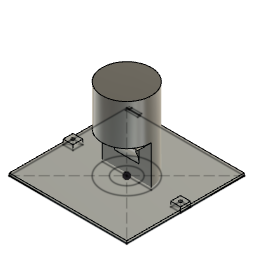
Minecraft Lamp (150x150mm) v6 (Autodesk Fusion 360 design; units mm, degrees)
Autodesk Fusion 360 part; units mm, degrees
sketch "Shade - Vertical Projection" plane through (0, 0, 0) normal (0, 0, 1) x (1, 0, 0) in component "Lamp Shade"
  line L0 (-75, 75) -> (75, 75)
  line L1 (75, 75) -> (75, -75)
  line L2 (75, -75) -> (-75, -75)
  line L3 (-75, -75) -> (-75, 75)
  line L4 (-75, 75) -> (75, -75) construction
  line L5 (75, 75) -> (-75, -75) construction
  line L6 (-72, 72) -> (72, 72)
  line L7 (72, 72) -> (72, -72)
  line L8 (72, -72) -> (-72, -72)
  line L9 (-72, -72) -> (-72, 72)
  line L10 (-72, 72) -> (72, -72) construction
  line L11 (72, 72) -> (-72, -72) construction
  line L12 (-66, 72) -> (-72, 72) construction
  line L13 (-72, 72) -> (-72, 75) construction
  line L14 (-72, 75) -> (-66, 75) construction
  line L15 (-66, 75) -> (-66, 72)
  line L16 (-75, 75) -> (-72, 75) construction
  line L17 (-72, 75) -> (-72, 72) construction
  line L18 (-72, 72) -> (-75, 72) construction
  line L19 (-75, 72) -> (-75, 75) construction
  line L20 (-54, 72) -> (-66, 72)
  line L21 (-66, 72) -> (-66, 75) construction
  line L22 (-66, 75) -> (-54, 75)
  line L23 (-54, 75) -> (-54, 72)
  line L24 (-72, 6) -> (-60, 6)
  line L25 (-60, 6) -> (-60, -6)
  line L26 (-60, -6) -> (-72, -6)
  line L27 (-72, -6) -> (-72, 6)
  line L28 (60, 6) -> (72, 6)
  line L29 (72, 6) -> (72, -6)
  line L30 (72, -6) -> (60, -6)
  line L31 (60, -6) -> (60, 6)
  dimension "d13" = 150
  dimension "d14" = 150
  dimension "d16" = 144
  dimension "d17" = 144
  dimension "d29" = 6
  dimension "d30" = 3
  dimension "d31" = 3
  dimension "d32" = 3
  dimension "d33" = 12
  dimension "d34" = 3
  dimension "d157" = 12
  dimension "d158" = 12
  dimension "d159" = 12
  dimension "d160" = 12
  constraint horizontal L0
  constraint perpendicular L0 L1
  constraint parallel L0 L2
  constraint parallel L1 L3
  constraint coincident L4 origin
  constraint coincident L5 origin
  constraint horizontal L6
  constraint perpendicular L6 L7
  constraint parallel L6 L8
  constraint parallel L7 L9
  constraint coincident L10 origin
  constraint coincident L11 origin
  constraint horizontal L12
  constraint vertical L13
  constraint horizontal L14
  constraint vertical L15
  constraint horizontal L16
  constraint vertical L17
  constraint horizontal L18
  constraint vertical L19
  constraint midpoint L13 L17
  constraint horizontal L20
  constraint vertical L21
  constraint horizontal L22
  constraint vertical L23
  constraint midpoint L15 L21
  constraint horizontal L24
  constraint vertical L25
  constraint horizontal L26
  constraint vertical L27
  constraint midpoint L9 L27
  constraint horizontal L28
  constraint vertical L29
  constraint horizontal L30
  constraint vertical L31
  constraint midpoint L7 L29
  measures "d13" distance of L1.end L2.end
  measures "d14" distance of L0.end L1.end
  measures "d16" distance of L7.end L8.end
  measures "d17" distance of L6.end L7.end
  measures "d29" distance of L12.start L6.start
  measures "d30" distance of L12.start L14.end
  measures "d31" distance of L0.start L13.end
  measures "d32" distance of L0.start L18.end
  measures "d33" distance of L20.start L12.start
  measures "d34" distance of L20.start L22.end
  measures "d157" distance of L24.start L24.end
  measures "d158" distance of L24.start L26.end
  measures "d159" distance of L28.start L28.end
  measures "d160" distance of L28.start L30.end
extrude "Extrude3" add sketch "Shade - Vertical Projection" along normal blind 150 contours L0 L1 L2 L3 L6 L7 L8 L9 L15 L23 L27 L29 | L0 L6 L15 L20 L22 L23 makes body 1 in component "Lamp Shade"
box "BoxPrimitive2" add length 150 width 150 height -3 placed x (0, 1, 0) y (-1, 0, 0) z (0, 0, 1) at (75, -75, 150) bodies 1 in component "Lamp Shade"
sketch "Shade - Back - Holes" plane through (0, 75, 0) normal (0, 1, 0) x (-1, 0, 0) in component "Lamp Shade"
  line L0 (-75, 150) -> (-75, 0)
  line L1 (-75, 0) -> (75, 0)
  line L2 (75, 0) -> (75, 150)
  line L3 (75, 150) -> (-75, 150)
  line L4 (75, 0) -> (69, 0)
  line L5 (69, 0) -> (69, 27) construction
  line L6 (69, 27) -> (75, 27) construction
  line L7 (75, 27) -> (75, 0)
  line L8 (69, 0) -> (57, 0)
  line L9 (57, 0) -> (57, 27)
  line L10 (57, 27) -> (69, 27) construction
  line L11 (69, 27) -> (69, 0)
  line L12 (57, 0) -> (30, 0)
  line L13 (30, 0) -> (30, 27) construction
  line L14 (30, 27) -> (57, 27) construction
  line L15 (57, 27) -> (57, 0) construction
  line L16 (69, 27) -> (57, 0) construction
  line L17 (69, 0) -> (57, 27) construction
  line L18 (57, 27) -> (30, 0) construction
  line L19 (30, 27) -> (57, 0) construction
  circle A0 centre (63, 13.5) radius 6
  circle A1 centre (43.5, 13.5) radius 7.5
  line L20 (69, 0) -> (57, 0)
  line L21 (57, 0) -> (57, 13.5)
  line L22 (57, 13.5) -> (69, 13.5)
  line L23 (69, 13.5) -> (69, 0)
  point P0 (75, 0)
  dimension "d61" = 6
  dimension "d62" = 27
  dimension "d63" = 12
  dimension "d64" = 27
  dimension "d65" = 27
  dimension "d66" = 27
  dimension "d67" = 12
  dimension "d68" = 15
  dimension "d69" = 12
  dimension "d70" = 13.5
  constraint horizontal L4
  constraint vertical L5
  constraint horizontal L6
  constraint vertical L7
  constraint coincident P0 L1.end
  constraint horizontal L8
  constraint vertical L9
  constraint horizontal L10
  constraint vertical L11
  constraint horizontal L12
  constraint vertical L13
  constraint horizontal L14
  constraint vertical L15
  constraint midpoint L17 A0.centre
  constraint midpoint L19 A1.centre
  constraint horizontal L20
  constraint vertical L21
  constraint horizontal L22
  constraint vertical L23
  constraint midpoint L8 L20
  measures "d61" distance of P0 L4.end
  measures "d62" distance of P0 L6.end
  measures "d63" distance of L4.end L8.end
  measures "d64" distance of L4.end L5.end
  measures "d65" distance of L8.end L12.end
  measures "d66" distance of L8.end L9.end
  measures "d67" diameter of A0
  measures "d68" diameter of A1
  measures "d69" distance of L4.end L8.end
  measures "d70" distance of L4.end L22.end
extrude "Extrude5" cut sketch "Shade - Back - Holes" against normal blind 3 contours L1 L8 L9 L11 A0 L20 L21 L23 | A0 L22 | A0 L22 | A1 bodies 1 in component "Lamp Shade"
sketch "Shade - Left" plane through (-75, 0, 0) normal (-1, 0, 0) x (0, -1, 0) in component "Lamp Shade"
  line L0 (-75, 150) -> (-75, 0)
  line L1 (-75, 0) -> (75, 0)
  line L2 (75, 0) -> (75, 150)
  line L3 (75, 150) -> (-75, 150)
  line L4 (-75, 150) -> (75, 150)
  line L5 (75, 150) -> (75, 0)
  line L6 (75, 0) -> (-75, 0)
  line L7 (-75, 0) -> (-75, 150)
  line L8 (75, 0) -> (-75, 0)
  line L9 (-64.2857, 0) -> (-64.2857, 150)
  line L10 (-53.5714, 0) -> (-53.5714, 150)
  line L11 (-42.8571, 0) -> (-42.8571, 150)
  line L12 (-32.1429, 0) -> (-32.1429, 150)
  line L13 (-21.4286, 0) -> (-21.4286, 150)
  line L14 (-10.7143, 0) -> (-10.7143, 150)
  line L15 (0, 0) -> (0, 150)
  line L16 (10.7143, 0) -> (10.7143, 150)
  line L17 (21.4286, 0) -> (21.4286, 150)
  line L18 (32.1429, 0) -> (32.1429, 150)
  line L19 (42.8571, 0) -> (42.8571, 150)
  line L20 (53.5714, 0) -> (53.5714, 150)
  line L21 (64.2857, 0) -> (64.2857, 150)
  line L22 (75, 0) -> (75, 150)
  line L23 (75, 10.7143) -> (-75, 10.7143)
  line L24 (75, 21.4286) -> (-75, 21.4286)
  line L25 (75, 32.1429) -> (-75, 32.1429)
  line L26 (75, 42.8571) -> (-75, 42.8571)
  line L27 (75, 53.5714) -> (-75, 53.5714)
  line L28 (75, 64.2857) -> (-75, 64.2857)
  line L29 (75, 75) -> (-75, 75)
  line L30 (75, 85.7143) -> (-75, 85.7143)
  line L31 (75, 96.4286) -> (-75, 96.4286)
  line L32 (75, 107.1429) -> (-75, 107.1429)
  line L33 (75, 117.8571) -> (-75, 117.8571)
  line L34 (75, 128.5714) -> (-75, 128.5714)
  line L35 (75, 139.2857) -> (-75, 139.2857)
  line L36 (75, 150) -> (-75, 150)
  dimension "d73" = 150
  dimension "d74" = 150
  dimension "d77" = 150
  dimension "d78" = 0
  dimension "d81" = 0
  dimension "d82" = 150
  constraint horizontal L4
  constraint vertical L5
  constraint horizontal L6
  constraint vertical L7
  constraint midpoint L6 L8
  measures "d73" distance of L0.start L2.end
  measures "d74" distance of L0.start L0.end
sketch "Shade - Front" plane through (0, -75, 0) normal (0, -1, 0) x (1, 0, 0) in component "Lamp Shade"
  line L0 (-75, 150) -> (-75, 0)
  line L1 (-75, 0) -> (75, 0)
  line L2 (75, 0) -> (75, 150)
  line L3 (75, 150) -> (-75, 150)
  line L4 (-75, 150) -> (75, 150)
  line L5 (75, 150) -> (75, 0)
  line L6 (75, 0) -> (-75, 0)
  line L7 (-75, 0) -> (-75, 150)
  line L8 (75, 0) -> (-75, 0)
  line L9 (75, 10.7143) -> (-75, 10.7143)
  line L10 (75, 21.4286) -> (-75, 21.4286)
  line L11 (75, 32.1429) -> (-75, 32.1429)
  line L12 (75, 42.8571) -> (-75, 42.8571)
  line L13 (75, 53.5714) -> (-75, 53.5714)
  line L14 (75, 64.2857) -> (-75, 64.2857)
  line L15 (75, 75) -> (-75, 75)
  line L16 (75, 85.7143) -> (-75, 85.7143)
  line L17 (75, 96.4286) -> (-75, 96.4286)
  line L18 (75, 107.1429) -> (-75, 107.1429)
  line L19 (75, 117.8571) -> (-75, 117.8571)
  line L20 (75, 128.5714) -> (-75, 128.5714)
  line L21 (75, 139.2857) -> (-75, 139.2857)
  line L22 (75, 150) -> (-75, 150)
  line L23 (-64.2857, 0) -> (-64.2857, 150)
  line L24 (-53.5714, 0) -> (-53.5714, 150)
  line L25 (-42.8571, 0) -> (-42.8571, 150)
  line L26 (-32.1429, 0) -> (-32.1429, 150)
  line L27 (-21.4286, 0) -> (-21.4286, 150)
  line L28 (-10.7143, 0) -> (-10.7143, 150)
  line L29 (0, 0) -> (0, 150)
  line L30 (10.7143, 0) -> (10.7143, 150)
  line L31 (21.4286, 0) -> (21.4286, 150)
  line L32 (32.1429, 0) -> (32.1429, 150)
  line L33 (42.8571, 0) -> (42.8571, 150)
  line L34 (53.5714, 0) -> (53.5714, 150)
  line L35 (64.2857, 0) -> (64.2857, 150)
  line L36 (75, 0) -> (75, 150)
  line L37 (-75, 150) -> (75, 0) construction
  line L38 (75, 150) -> (-75, 0) construction
  dimension "d83" = 150
  dimension "d84" = 150
  dimension "d87" = 0
  dimension "d88" = 150
  dimension "d91" = 150
  dimension "d92" = 0
  constraint horizontal L4
  constraint vertical L5
  constraint horizontal L6
  constraint vertical L7
  constraint midpoint L6 L8
  constraint coincident L1.end L2.start
  constraint coincident L0.end L1.start
  measures "d83" distance of L0.start L2.end
  measures "d84" distance of L0.start L0.end
sketch "Shade - Right" plane through (75, 0, 0) normal (1, 0, 0) x (0, 1, 0) in component "Lamp Shade"
  line L0 (-75, 150) -> (-75, 0)
  line L1 (-75, 0) -> (75, 0)
  line L2 (75, 0) -> (75, 150)
  line L3 (75, 150) -> (-75, 150)
  line L4 (-75, 150) -> (75, 150)
  line L5 (75, 150) -> (75, 0)
  line L6 (75, 0) -> (-75, 0)
  line L7 (-75, 0) -> (-75, 150)
  line L8 (75, 0) -> (-75, 0)
  line L9 (-64.2857, 0) -> (-64.2857, 150)
  line L10 (-53.5714, 0) -> (-53.5714, 150)
  line L11 (-42.8571, 0) -> (-42.8571, 150)
  line L12 (-32.1429, 0) -> (-32.1429, 150)
  line L13 (-21.4286, 0) -> (-21.4286, 150)
  line L14 (-10.7143, 0) -> (-10.7143, 150)
  line L15 (0, 0) -> (0, 150)
  line L16 (10.7143, 0) -> (10.7143, 150)
  line L17 (21.4286, 0) -> (21.4286, 150)
  line L18 (32.1429, 0) -> (32.1429, 150)
  line L19 (42.8571, 0) -> (42.8571, 150)
  line L20 (53.5714, 0) -> (53.5714, 150)
  line L21 (64.2857, 0) -> (64.2857, 150)
  line L22 (75, 0) -> (75, 150)
  line L23 (75, 10.7143) -> (-75, 10.7143)
  line L24 (75, 21.4286) -> (-75, 21.4286)
  line L25 (75, 32.1429) -> (-75, 32.1429)
  line L26 (75, 42.8571) -> (-75, 42.8571)
  line L27 (75, 53.5714) -> (-75, 53.5714)
  line L28 (75, 64.2857) -> (-75, 64.2857)
  line L29 (75, 75) -> (-75, 75)
  line L30 (75, 85.7143) -> (-75, 85.7143)
  line L31 (75, 96.4286) -> (-75, 96.4286)
  line L32 (75, 107.1429) -> (-75, 107.1429)
  line L33 (75, 117.8571) -> (-75, 117.8571)
  line L34 (75, 128.5714) -> (-75, 128.5714)
  line L35 (75, 139.2857) -> (-75, 139.2857)
  line L36 (75, 150) -> (-75, 150)
  dimension "d93" = 150
  dimension "d94" = 150
  dimension "d97" = 150
  dimension "d98" = 0
  dimension "d101" = 0
  dimension "d102" = 150
  constraint horizontal L4
  constraint vertical L5
  constraint horizontal L6
  constraint vertical L7
  constraint midpoint L6 L8
  measures "d93" distance of L0.start L2.end
  measures "d94" distance of L0.start L0.end
sketch "Shade - Back" plane through (0, 75, 0) normal (0, 1, 0) x (-1, 0, 0) in component "Lamp Shade"
  line L0 (57, 0) -> (57, 13.5)
  arc A0 (69, 13.5) -> (57, 13.5) centre (63, 13.5) ccw
  line L1 (69, 13.5) -> (69, 0)
  line L2 (69, 0) -> (75, 0)
  line L3 (75, 0) -> (75, 150)
  line L4 (75, 150) -> (-75, 150)
  line L5 (-75, 150) -> (-75, 0)
  line L6 (-75, 0) -> (57, 0)
  circle A1 centre (43.5, 13.5) radius 7.5
  line L7 (-75, 150) -> (75, 150)
  line L8 (75, 150) -> (75, 0)
  line L9 (75, 0) -> (-75, 0)
  line L10 (-75, 0) -> (-75, 150)
  line L11 (75, 0) -> (-75, 0)
  line L12 (75, 10.7143) -> (-75, 10.7143)
  line L13 (75, 21.4286) -> (-75, 21.4286)
  line L14 (75, 32.1429) -> (-75, 32.1429)
  line L15 (75, 42.8571) -> (-75, 42.8571)
  line L16 (75, 53.5714) -> (-75, 53.5714)
  line L17 (75, 64.2857) -> (-75, 64.2857)
  line L18 (75, 75) -> (-75, 75)
  line L19 (75, 85.7143) -> (-75, 85.7143)
  line L20 (75, 96.4286) -> (-75, 96.4286)
  line L21 (75, 107.1429) -> (-75, 107.1429)
  line L22 (75, 117.8571) -> (-75, 117.8571)
  line L23 (75, 128.5714) -> (-75, 128.5714)
  line L24 (75, 139.2857) -> (-75, 139.2857)
  line L25 (75, 150) -> (-75, 150)
  line L26 (-64.2857, 0) -> (-64.2857, 150)
  line L27 (-53.5714, 0) -> (-53.5714, 150)
  line L28 (-42.8571, 0) -> (-42.8571, 150)
  line L29 (-32.1429, 0) -> (-32.1429, 150)
  line L30 (-21.4286, 0) -> (-21.4286, 150)
  line L31 (-10.7143, 0) -> (-10.7143, 150)
  line L32 (0, 0) -> (0, 150)
  line L33 (10.7143, 0) -> (10.7143, 150)
  line L34 (21.4286, 0) -> (21.4286, 150)
  line L35 (32.1429, 0) -> (32.1429, 150)
  line L36 (42.8571, 0) -> (42.8571, 150)
  line L37 (53.5714, 0) -> (53.5714, 150)
  line L38 (64.2857, 0) -> (64.2857, 150)
  line L39 (75, 0) -> (75, 150)
  dimension "d103" = 150
  dimension "d104" = 150
  dimension "d107" = 0
  dimension "d108" = 150
  dimension "d111" = 150
  dimension "d112" = 0
  constraint horizontal L7
  constraint vertical L8
  constraint horizontal L9
  constraint vertical L10
  constraint midpoint L9 L11
  measures "d103" distance of L4.end L3.end
  measures "d104" distance of L4.end L5.end
sketch "Shade - Top" plane through (0, 0, 150) normal (0, 0, 1) x (-1, 0, 0) in component "Lamp Shade"
  line L0 (75, 75) -> (-75, 75)
  line L1 (-75, 75) -> (-75, -75)
  line L2 (-75, -75) -> (75, -75)
  line L3 (75, -75) -> (75, 75)
  line L4 (-75, -75) -> (75, -75)
  line L5 (75, -75) -> (75, 75)
  line L6 (75, 75) -> (-75, 75)
  line L7 (-75, 75) -> (-75, -75)
  line L8 (75, 75) -> (-75, 75)
  line L9 (-64.2857, 75) -> (-64.2857, -75)
  line L10 (-53.5714, 75) -> (-53.5714, -75)
  line L11 (-42.8571, 75) -> (-42.8571, -75)
  line L12 (-32.1429, 75) -> (-32.1429, -75)
  line L13 (-21.4286, 75) -> (-21.4286, -75)
  line L14 (-10.7143, 75) -> (-10.7143, -75)
  line L15 (0, 75) -> (0, -75)
  line L16 (10.7143, 75) -> (10.7143, -75)
  line L17 (21.4286, 75) -> (21.4286, -75)
  line L18 (32.1429, 75) -> (32.1429, -75)
  line L19 (42.8571, 75) -> (42.8571, -75)
  line L20 (53.5714, 75) -> (53.5714, -75)
  line L21 (64.2857, 75) -> (64.2857, -75)
  line L22 (75, 75) -> (75, -75)
  line L23 (75, 64.2857) -> (-75, 64.2857)
  line L24 (75, 53.5714) -> (-75, 53.5714)
  line L25 (75, 42.8571) -> (-75, 42.8571)
  line L26 (75, 32.1429) -> (-75, 32.1429)
  line L27 (75, 21.4286) -> (-75, 21.4286)
  line L28 (75, 10.7143) -> (-75, 10.7143)
  line L29 (75, 0) -> (-75, 0)
  line L30 (75, -10.7143) -> (-75, -10.7143)
  line L31 (75, -21.4286) -> (-75, -21.4286)
  line L32 (75, -32.1429) -> (-75, -32.1429)
  line L33 (75, -42.8571) -> (-75, -42.8571)
  line L34 (75, -53.5714) -> (-75, -53.5714)
  line L35 (75, -64.2857) -> (-75, -64.2857)
  line L36 (75, -75) -> (-75, -75)
  dimension "d113" = 150
  dimension "d114" = 150
  dimension "d117" = 150
  dimension "d118" = 0
  dimension "d121" = 0
  constraint horizontal L4
  constraint vertical L5
  constraint horizontal L6
  constraint vertical L7
  constraint midpoint L6 L8
  measures "d113" distance of L1.end L2.end
  measures "d114" distance of L1.end L0.end
sketch "Base - Vertical Projection" plane through (0, 0, 0) normal (0, 0, 1) x (1, 0, 0) in component "Lamp Base"
  line L0 (-72, 72) -> (72, 72)
  line L1 (72, 72) -> (72, -72)
  line L2 (72, -72) -> (-72, -72)
  line L3 (-72, -72) -> (-72, 72)
  line L4 (-72, 72) -> (72, -72) construction
  line L5 (72, 72) -> (-72, -72) construction
  line L6 (-72, 72) -> (-69, 72)
  line L7 (-69, 72) -> (-69, 75)
  line L8 (-69, 75) -> (-72, 75) construction
  line L9 (-72, 75) -> (-72, 72) construction
  line L10 (-57, 72) -> (-69, 72)
  line L11 (-69, 72) -> (-69, 75)
  line L12 (-69, 75) -> (-57, 75)
  line L13 (-57, 75) -> (-57, 72)
  line L14 (-55.5, 69) -> (-70.5, 69)
  line L15 (-70.5, 69) -> (-70.5, 72)
  line L16 (-70.5, 72) -> (-55.5, 72)
  line L17 (-55.5, 72) -> (-55.5, 69)
  line L18 (-60, -6) -> (-72, -6)
  line L19 (-72, -6) -> (-72, 6)
  line L20 (-72, 6) -> (-60, 6)
  line L21 (-60, 6) -> (-60, -6)
  line L22 (72, -6) -> (60, -6)
  line L23 (60, -6) -> (60, 6)
  line L24 (60, 6) -> (72, 6)
  line L25 (72, 6) -> (72, -6)
  line L26 (-60, -6) -> (-72, 6) construction
  line L27 (-72, -6) -> (-60, 6) construction
  line L28 (60, -6) -> (72, 6) construction
  line L29 (72, -6) -> (60, 6) construction
  circle A0 centre (0, 0) radius 30
  circle A1 centre (0, 0) radius 15
  line L30 (0, 0) -> (-30, 0)
  line L31 (0, 0) -> (30, 0)
  dimension "d123" = 144
  dimension "d124" = 144
  dimension "d125" = 3
  dimension "d126" = 3
  dimension "d127" = 12
  dimension "d128" = 3
  dimension "d129" = 15
  dimension "d130" = 3
  dimension "d131" = 12
  dimension "d132" = 12
  dimension "d133" = 12
  dimension "d134" = 12
  dimension "d154" = 60
  dimension "d176" = 30
  constraint horizontal L0
  constraint perpendicular L0 L1
  constraint parallel L0 L2
  constraint parallel L1 L3
  constraint coincident L4 A0.centre
  constraint coincident L5 A0.centre
  constraint coincident A0.centre A1.centre
  constraint horizontal L6
  constraint vertical L7
  constraint horizontal L8
  constraint vertical L9
  constraint horizontal L10
  constraint vertical L11
  constraint horizontal L12
  constraint vertical L13
  constraint midpoint L7 L11
  constraint horizontal L14
  constraint vertical L15
  constraint horizontal L16
  constraint vertical L17
  constraint midpoint L10 L16
  constraint horizontal L18
  constraint vertical L19
  constraint horizontal L20
  constraint vertical L21
  constraint midpoint L3 L19
  constraint horizontal L22
  constraint vertical L23
  constraint horizontal L24
  constraint vertical L25
  constraint midpoint L1 L25
  constraint concentric A0 A1
  constraint coincident A0 L30.end
  constraint horizontal L30
  constraint coincident A0 L31.end
  constraint parallel L30 L31
  measures "d123" distance of L1.end L2.end
  measures "d124" distance of L0.end L1.end
  measures "d125" distance of L0.start L6.end
  measures "d126" distance of L0.start L8.end
  measures "d127" distance of L10.start L6.end
  measures "d128" distance of L10.start L12.end
  measures "d129" distance of L14.start L14.end
  measures "d130" distance of L14.start L16.end
  measures "d131" distance of L18.start L18.end
  measures "d132" distance of L18.start L20.end
  measures "d133" distance of L22.start L22.end
  measures "d134" distance of L22.start L24.end
  measures "d154" diameter of A0
  measures "d176" diameter of A1
extrude "Extrude1" add sketch "Base - Vertical Projection" along normal blind 3 separate body contours L0 L1 L2 L3 L6 L14 L15 L17 L18 L20 L21 L22 L23 L24 | L0 L6 L10 L14 L15 L16 L17 | L3 L18 L19 L20 L21 | L1 L22 L23 L24 L25 | A0 A1 L30 L31 | A0 A1 L30 L31 | A1 L30 L31 | A1 L30 L31 makes body 2 in component "Lamp Base"
sketch "Base - Back - Holes" plane through (0, 72, 0) normal (0, 1, 0) x (-1, 0, 0) in component "Lamp Base"
  line L0 (-72, 0) -> (72, 0)
  line L1 (72, 0) -> (72, 3)
  line L2 (72, 3) -> (-72, 3)
  line L3 (-72, 3) -> (-72, 0)
  line L4 (57, 13.5, 3) -> (69, 13.5, 3)
  line L5 (69, 13.5, 3) -> (69, 0, 3)
  line L6 (69, 0, 3) -> (57, 0, 3)
  line L7 (57, 0, 3) -> (57, 13.5, 3)
  line L8 (69, 0, 3) -> (57, 0, 3)
  circle A0 through (69, 13.5, 3) (60, 18.6962, 3) (60, 8.3038, 3)
  line L9 (55.5, 0) -> (70.5, 0)
  line L10 (70.5, 0) -> (70.5, 15)
  line L11 (70.5, 15) -> (55.5, 15)
  line L12 (55.5, 15) -> (55.5, 0)
  line L13 (70.5, 0) -> (55.5, 0) construction
  circle A1 centre (63, 15) radius 7.5
  dimension "d140" = 12
  dimension "d141" = 13.5
  dimension "d142" = 12
  dimension "d144" = 15
  dimension "d145" = 15
  dimension "d146" = 15
  constraint horizontal L9
  constraint vertical L10
  constraint horizontal L11
  constraint vertical L12
  constraint midpoint L9 L13
  constraint midpoint L11 A1.centre
  measures "d144" distance of L9.start L9.end
  measures "d145" distance of L9.start L11.end
  measures "d146" diameter of A1
extrude "Extrude2" add sketch "Base - Back - Holes" against normal blind 3 separate body contours L4 A0 | L5 L6 L7 L8 A0 | L4 A0 in plane through (0, 75, 0) normal (0, 1, 0) makes body 3 in component "Lamp Base"
extrude "Extrude3'" add sketch "Base - Back - Holes" against normal blind 3 contours L0 L2 L9 L10 L12 | L2 L10 L12 A1 | L11 A1 | L11 A1 bodies 3 in component "Lamp Base"
hole "Hole1" at (-63, 75, 13.5) direction (0, -1, 0) diameter 5 end up to surface (6 mm away) bodies 3 in component "Lamp Base"
extrude "Extrude4" add sketch "Base - Vertical Projection" along normal blind 6 separate body contours L3 L18 L19 L20 L21 | L1 L22 L23 L24 L25 makes body 4 at (64, 2, 0) makes body 5 at (-68, 2, 0) in component "Lamp Base"
extrude "Extrude6" add sketch "Shade - Vertical Projection" along normal blind 6 from surface at 6 separate body contours L9 L24 L25 L26 L27 | L7 L28 L29 L30 L31 makes body 6 at (-68, 2, 6) makes body 7 at (64, 2, 6) in component "Lamp Shade"
hole "Hole1'" at (66, 0, 0) direction (0, 0, 1) diameter 3.8 depth 9 tip angle 90 bodies 7 in component "Lamp Shade"
hole "Hole2" at (66, 0, 0) direction (0, 0, 1) diameter 3.8 depth 9 tip angle 90 bodies 2 4 in component "Lamp Base"
hole "Hole2'" at (-66, 0, 0) direction (0, 0, 1) diameter 3.8 depth 9 tip angle 90 bodies 6 in component "Lamp Shade"
hole "Hole3" at (-66, 0, 0) direction (0, 0, 1) diameter 3.8 depth 9 tip angle 90 bodies 2 5 in component "Lamp Base"
extrude "Extrude6'" add sketch "Base - Vertical Projection" along normal blind 50 separate body contours A1 L30 L31 picked at (-9.9442, 0.7452) makes body 8 in component "Lamp Base"
extrude "Extrude7" add sketch "Base - Vertical Projection" along normal blind 50 from surface at 50 contours A0 A1 L30 L31 | A0 A1 L30 L31 | A1 L30 L31 | A1 L30 L31 bodies 8 in component "Lamp Base"
chamfer "Chamfer1" distance 15 angle 45 1 edges at (0, 15, 50) on bodies 8 in component "Lamp Base"
fillet "Fillet1" radius 30 1 edges at (0, 0, 50) on bodies 8 in component "Lamp Base"
extrude "Extrude8" add sketch "Base - Vertical Projection" along normal blind 50 contours A0 A1 L30 L31 picked at (-19.2582, 15.8358) bodies 8 in component "Lamp Base"
sketch "Sketch12" plane through (0, -72, 0) normal (0, 1, 0) x (-1, 0, 0) in component "Lamp Difusser"
  line L0 (72, 147) -> (-72, 147)
  line L1 (-72, 147) -> (-72, 0)
  line L2 (-72, 0) -> (72, 0)
  line L3 (72, 0) -> (72, 147)
  line L4 (-70.5, 145.5, -3) -> (70.5, 145.5, -3)
  line L5 (70.5, 145.5, -3) -> (70.5, 4.5, -3)
  line L6 (70.5, 4.5, -3) -> (-70.5, 4.5, -3)
  line L7 (-70.5, 4.5, -3) -> (-70.5, 145.5, -3)
  line L8 (-70.5, 145.5, -3) -> (70.5, 4.5, -3) construction
  line L9 (70.5, 145.5, -3) -> (-70.5, 4.5, -3) construction
  line L10 (0, 0, -3) -> (0, 150, -3)
  point P0 (0, 75)
  dimension "d192" = 141
  dimension "d193" = 141
extrude "Extrude2'" add sketch "Sketch12" along normal blind 0.5 separate body makes body 9 in component "Lamp Difusser"
extrude "Extrude7'" cut sketch "Shade - Top" against normal blind 3 contours L18 L19 L23 L24 | L19 L20 L24 L25 | L18 L19 L24 L25 | L20 L21 L26 L27 | L19 L20 L26 L27 | L15 L16 L23 L24 | L18 L19 L26 L27 | L19 L20 L27 L28 | L14 L15 L23 L24 | L18 L19 L27 L28 | L14 L15 L24 L25 | L20 L21 L30 L31 | L13 L14 L24 L25 | L14 L15 L25 L26 | L19 L20 L30 L31 | L12 L13 L24 L25 | L13 L14 L25 L26 | L18 L19 L30 L31 | L20 L21 L32 L33 | L12 L13 L25 L26 | L17 L18 L30 L31 | L19 L20 L32 L33 | L20 L21 L33 L34 | L9 L10 L23 L24 | L11 L12 L25 L26 | L14 L15 L28 L29 | L16 L17 L30 L31 | L17 L18 L31 L32 | L19 L20 L33 L34 | L10 L11 L25 L26 | L11 L12 L26 L27 | L13 L14 L28 L29 | L14 L15 L29 L30 | L16 L17 L31 L32 | L19 L20 L34 L35 | L9 L10 L25 L26 | L10 L11 L26 L27 | L12 L13 L28 L29 | L13 L14 L29 L30 | L16 L17 L33 L34 | L15 L16 L33 L34 | L12 L13 L31 L32 | L14 L15 L33 L34 | L9 L10 L29 L30 | L11 L12 L31 L32 | L12 L13 L32 L33 | L11 L12 L32 L33 | L10 L11 L34 L35 | L9 L10 L34 L35 bodies 1 in component "Lamp Shade"
extrude "Extrude8'" cut sketch "Shade - Back" against normal blind 3 contours L14 L15 L35 L36 | L15 L16 L37 L38 | L15 L16 L36 L37 | L12 L13 L33 L34 | L13 L14 L33 L34 | L15 L16 L35 L36 | L12 L13 L32 L33 | L13 L14 L32 L33 | L15 L16 L34 L35 | L15 L16 L33 L34 | L17 L18 L35 L36 | L18 L19 L37 L38 | L18 L19 L36 L37 | L15 L16 L32 L33 | L18 L19 L35 L36 | L13 L14 L29 L30 | L16 L17 L32 L33 | L13 L14 L28 L29 | L17 L18 L32 L33 | L21 L22 L37 L38 | L13 L14 L27 L28 | L14 L15 L28 L29 | L17 L18 L31 L32 | L21 L22 L35 L36 | L22 L23 L37 L38 | L22 L23 L36 L37 | L13 L14 L26 L27 | L14 L15 L27 L28 | L18 L19 L31 L32 | L22 L23 L35 L36 | L14 L15 L26 L27 | L16 L17 L28 L29 | L20 L21 L32 L33 | L23 L24 L35 L36 | L17 L18 L28 L29 | L16 L17 L26 L27 | L18 L19 L28 L29 | L18 L19 L27 L28 | L22 L23 L30 L31 | L22 L23 L29 L30 | L21 L22 L27 L28 | L23 L24 L29 L30 | L21 L22 L26 L27 | L23 L24 L28 L29 | L23 L24 L27 L28 bodies 1 in component "Lamp Shade"
extrude "Extrude9" cut sketch "Shade - Left" against normal blind 3 contours L9 L10 L32 L33 | L10 L11 L33 L34 | L9 L10 L31 L32 | L10 L11 L32 L33 | L10 L11 L31 L32 | L10 L11 L30 L31 | L11 L12 L31 L32 | L13 L14 L33 L34 | L10 L11 L29 L30 | L13 L14 L32 L33 | L14 L15 L32 L33 | L9 L10 L26 L27 | L14 L15 L31 L32 | L15 L16 L32 L33 | L9 L10 L25 L26 | L15 L16 L31 L32 | L10 L11 L25 L26 | L12 L13 L27 L28 | L16 L17 L31 L32 | L19 L20 L34 L35 | L10 L11 L24 L25 | L13 L14 L27 L28 | L14 L15 L28 L29 | L17 L18 L31 L32 | L20 L21 L34 L35 | L11 L12 L24 L25 | L14 L15 L27 L28 | L20 L21 L33 L34 | L12 L13 L24 L25 | L14 L15 L26 L27 | L16 L17 L28 L29 | L17 L18 L29 L30 | L17 L18 L28 L29 | L19 L20 L29 L30 | L15 L16 L24 L25 | L19 L20 L28 L29 | L20 L21 L29 L30 | L16 L17 L24 L25 | L20 L21 L28 L29 | L17 L18 L24 L25 | L18 L19 L25 L26 | L19 L20 L26 L27 | L18 L19 L24 L25 | L19 L20 L25 L26 | L20 L21 L25 L26 bodies 1 in component "Lamp Shade"
extrude "Extrude10" cut sketch "Shade - Front" against normal blind 3 contours L19 L20 L24 L25 | L17 L18 L23 L24 | L19 L20 L25 L26 | L17 L18 L24 L25 | L18 L19 L25 L26 | L17 L18 L25 L26 | L14 L15 L23 L24 | L13 L14 L23 L24 | L14 L15 L24 L25 | L15 L16 L25 L26 | L18 L19 L28 L29 | L19 L20 L29 L30 | L13 L14 L24 L25 | L14 L15 L25 L26 | L17 L18 L28 L29 | L18 L19 L29 L30 | L19 L20 L30 L31 | L14 L15 L26 L27 | L16 L17 L28 L29 | L18 L19 L30 L31 | L16 L17 L29 L30 | L11 L12 L25 L26 | L19 L20 L33 L34 | L10 L11 L25 L26 | L19 L20 L34 L35 | L10 L11 L26 L27 | L11 L12 L27 L28 | L14 L15 L30 L31 | L10 L11 L27 L28 | L16 L17 L33 L34 | L17 L18 L34 L35 | L9 L10 L27 L28 | L16 L17 L34 L35 | L9 L10 L28 L29 | L12 L13 L31 L32 | L15 L16 L34 L35 | L11 L12 L31 L32 | L12 L13 L32 L33 | L14 L15 L34 L35 | L10 L11 L31 L32 | L13 L14 L34 L35 | L10 L11 L32 L33 bodies 1 in component "Lamp Shade"
extrude "Extrude11" cut sketch "Shade - Right" against normal blind 3 contours L9 L10 L33 L34 | L10 L11 L33 L34 | L10 L11 L32 L33 | L11 L12 L32 L33 | L14 L15 L33 L34 | L9 L10 L27 L28 | L10 L11 L28 L29 | L14 L15 L32 L33 | L15 L16 L33 L34 | L9 L10 L26 L27 | L10 L11 L27 L28 | L12 L13 L29 L30 | L13 L14 L30 L31 | L17 L18 L34 L35 | L9 L10 L25 L26 | L11 L12 L27 L28 | L17 L18 L33 L34 | L10 L11 L25 L26 | L17 L18 L32 L33 | L18 L19 L33 L34 | L15 L16 L29 L30 | L19 L20 L33 L34 | L13 L14 L26 L27 | L14 L15 L27 L28 | L16 L17 L29 L30 | L19 L20 L32 L33 | L12 L13 L24 L25 | L14 L15 L26 L27 | L16 L17 L28 L29 | L17 L18 L29 L30 | L12 L13 L23 L24 | L14 L15 L25 L26 | L15 L16 L26 L27 | L17 L18 L28 L29 | L19 L20 L30 L31 | L15 L16 L25 L26 | L15 L16 L24 L25 | L20 L21 L28 L29 | L19 L20 L26 L27 | L20 L21 L27 L28 | L18 L19 L24 L25 | L19 L20 L25 L26 | L20 L21 L26 L27 | L19 L20 L24 L25 bodies 1 in component "Lamp Shade"
extrude "Extrude1'" [suppressed] in component "Lamp Difusser"
component "Minecraft Lamp" placed x (1, 0, 0) y (0, 1, 0) z (0, 0, 1) at (0, 0, 0)
component "Lamp Shade" placed x (1, 0, 0) y (0, 1, 0) z (0, 0, 1) at (0, 0, 0) in component "Minecraft Lamp"
component "Lamp Base" placed x (1, 0, 0) y (0, 1, 0) z (0, 0, 1) at (0, 0, 0) in component "Minecraft Lamp"
component "Lamp Difusser" placed x (1, 0, 0) y (0, 1, 0) z (0, 0, 1) at (0, 0, 0) in component "Minecraft Lamp"
component "Lamp Shade - Holes Example (15x15)" placed x (1, 0, 0) y (0, 1, 0) z (0, 0, 1) at (0, 0, 0) in component "Minecraft Lamp"
component "Lamp Shade" placed x (1, 0, 0) y (0, 1, 0) z (0, 0, 1) at (0, 0, 0.01) in component "Lamp Shade - Holes Example (15x15)"
hidden bodies 6 7
equation "sideLength = 150 mm" comment "Same for the external length, width and height"
equation "d13 = sideLength"
equation "d14 = sideLength"
equation "thickness = 3 mm" comment "3mm is robust enough, but feel free to modify it"
equation "d16 = sideLength - ( thickness * 2 )"
equation "d17 = sideLength - ( thickness * 2 )"
equation "d20 = sideLength"
equation "d24 = -thickness"
equation "d29 = thickness * 2"
equation "d30 = thickness"
equation "d31 = thickness"
equation "d32 = thickness"
equation "d33 = cordExternalDiameter"
equation "d34 = thickness"
equation "buttonDiameter = 15 mm" comment "Diameter of the pushbutton"
equation "cordExternalDiameter = 12 mm" comment "Diameter/length of the cord extrusion"
equation "sidePixels = 15" comment "Number of horizontal and vertical pixels for every side of the shade"
equation "d61 = thickness * 2"
equation "d62 = buttonDiameter + thickness * 4"
equation "d63 = cordExternalDiameter"
equation "d64 = buttonDiameter + thickness * 4"
equation "d65 = buttonDiameter + thickness * 4"
equation "d66 = buttonDiameter + thickness * 4"
equation "d67 = cordExternalDiameter"
equation "d68 = buttonDiameter"
equation "d69 = cordExternalDiameter"
equation "d70 = ( buttonDiameter + thickness * 4 ) / 2"
equation "d71 = -thickness"
equation "d73 = sideLength"
equation "d74 = sideLength"
equation "d75 = sidePixels"
equation "d77 = sideLength"
equation "d80 = sidePixels"
equation "d82 = sideLength"
equation "d83 = sideLength"
equation "d84 = sideLength"
equation "d86 = sidePixels"
equation "d88 = sideLength"
equation "d89 = sidePixels"
equation "d91 = sideLength"
equation "d93 = sideLength"
equation "d94 = sideLength"
equation "d95 = sidePixels"
equation "d97 = sideLength"
equation "d100 = sidePixels"
equation "d102 = sideLength"
equation "d103 = sideLength"
equation "d104 = sideLength"
equation "d106 = sidePixels"
equation "d108 = sideLength"
equation "d109 = sidePixels"
equation "d111 = sideLength"
equation "d113 = sideLength"
equation "d114 = sideLength"
equation "d115 = sidePixels"
equation "d117 = sideLength"
equation "d120 = sidePixels"
equation "d122 = -sideLength"
equation "d123 = sideLength - thickness * 2"
equation "d124 = sideLength - thickness * 2"
equation "d125 = thickness"
equation "d126 = thickness"
equation "d127 = cordExternalDiameter"
equation "d128 = thickness"
equation "d129 = cordExternalDiameter + thickness"
equation "d130 = thickness"
equation "M4Diameter = 3.8 mm" comment "Used at the 2 bottom holes"
equation "d138 = thickness"
equation "d140 = cordExternalDiameter"
equation "d141 = ( buttonDiameter + thickness * 4 ) / 2"
equation "d142 = cordExternalDiameter"
equation "cordDiameter = 5 mm" comment "Fits a regular USB cable"
equation "d144 = cordExternalDiameter + thickness"
equation "d145 = cordExternalDiameter + thickness"
equation "d146 = cordExternalDiameter + thickness"
equation "d147 = -thickness"
equation "d149 = -thickness"
equation "d152 = cordDiameter"
equation "d154 = ( sideLength / 5 ) * 2"
equation "d155 = thickness * 2"
equation "d161 = 2 * thickness"
equation "d162 = 2 * thickness"
equation "d164 = 3 * thickness"
equation "d165 = M4Diameter"
equation "d167 = 3 * thickness"
equation "d168 = M4Diameter"
equation "d170 = 3 * thickness"
equation "d171 = M4Diameter"
equation "d173 = 3 * thickness"
equation "d174 = M4Diameter"
equation "d176 = sideLength / 5"
equation "d179 = 1 / 3 * sideLength"
equation "d181 = 1 / 3 * sideLength"
equation "d182 = 1 / 3 * sideLength"
equation "d184 = 1 / 10 * sideLength"
equation "d185 = 1 / 5 * sideLength"
equation "d186 = 1 / 3 * sideLength"
equation "d192 = sideLength - ( thickness * 3 )"
equation "d193 = sideLength - ( thickness * 3 )"
equation "d196 = -thickness"
equation "d198 = -thickness"
equation "d200 = -thickness"
equation "d202 = -thickness"
equation "d204 = -thickness"
named bodies: "Lamp Shade", "Lamp Base", "Lamp Base - Back Holes", "Lamp Base - Right Support", "Lamp Base - Left Support", "Lamp Shade - Left Support", "Lamp Shade - Right Support", "Lamp Difusser"
